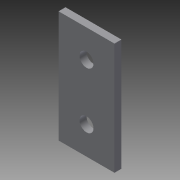
# Autodesk Inventor part: 2 hole plate
Saved by Autodesk Inventor 2014 (Build 180170000, 170)
## iProperties
Created: 2014-01-06
Part Number: 2 hole plate
Material: Generic
Document SubType Name: Modeling
Designer: Tristan Debrunner
Density: 1 g/cm^3
Appearance: Default
Author: Tristan Debrunner
Autodesk Inventor part; units mm, degrees
ref_plane "YZ Plane" through (0, 0, 0) normal (1, 0, 0) x (0, 1, 0)
ref_plane "XZ Plane" through (0, 0, 0) normal (0, 1, 0) x (-1, 0, 0)
ref_plane "XY Plane" through (0, 0, 0) normal (0, 0, 1) x (1, 0, 0)
sketch "Sketch1" plane through (0, 0, 0) normal (0, 0, 1) x (1, 0, 0)
  line L0 (-12.7, -25.4) -> (12.7, -25.4)
  line L1 (12.7, -25.4) -> (12.7, 25.4)
  line L2 (12.7, 25.4) -> (-12.7, 25.4)
  line L3 (-12.7, 25.4) -> (-12.7, -25.4)
  line L4 (-12.7, -25.4) -> (12.7, 25.4) construction
  line L5 (12.7, -25.4) -> (-12.7, 25.4) construction
  point P0 (0, 0)
  dimension "d0" = 25.4
  dimension "d1" = 50.8
  constraints: 12 end point, 2 midpoint, 2 parallel, 1 horizontal, 1 perpendicular
  measures "d0" distance of L2.end L1.end
  measures "d1" distance of L1.end L0.end
extrude "Extrusion1" add sketch "Sketch1" along normal blind 3.175
sketch "Sketch2" plane through (0, 0, 3.175) normal (0, 0, 1) x (1, 0, 0)
  line L0 (-12.7, -25.4) -> (12.7, -25.4) projected
  line L1 (12.7, 25.4) -> (-12.7, 25.4) projected
  line L2 (-12.7, 25.4) -> (-12.7, -25.4) projected
  line L3 (0, 25.4) -> (0, 12.7)
  line L4 (0, -25.4) -> (0, -12.7)
  point P0 (0, 0)
  dimension "d4" = 12.7
  dimension "d5" = 12.7
  constraints: 4 end point, 2 midpoint, 1 collinear, 1 parallel
  measures "d4" distance of L3.start L3.end
  measures "d5" distance of L4.start L4.end
hole "Hole1" at (0, 12.7, 3.175) at (0, -12.7, 3.175) direction (0, 0, -1) diameter 6.35 end through all
body "Solid1"
